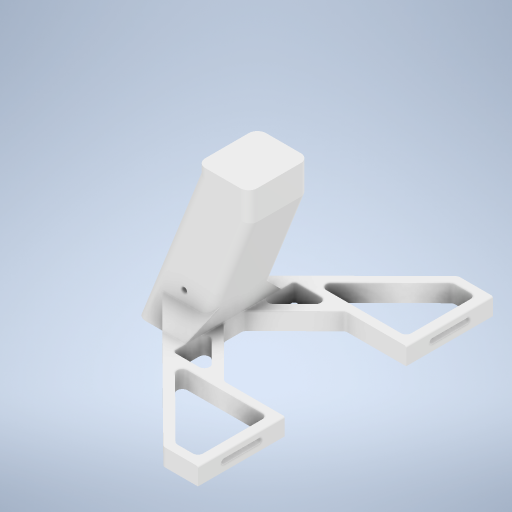
# Autodesk Inventor part: UpperLandingLegMount - BranchBrace+Shortened
Saved by Autodesk Inventor 2023 (Build 270158000, 158)
## iProperties
Created: 2023-01-11
Part Number: UpperLandingLegMount - BranchBrace+Shortened
Material: ABS Plastic
Document SubType Name: Modeling
Designer: chase
Density: 1.06 g/cm^3
Appearance: Smooth - White
Author: chase
Autodesk Inventor part; units mm, degrees
ref_plane "YZ Plane" through (0, 0, 0) normal (1, 0, 0) x (0, 1, 0)
ref_plane "XZ Plane" through (0, 0, 0) normal (0, 1, 0) x (-1, 0, 0)
ref_plane "XY Plane" through (0, 0, 0) normal (0, 0, 1) x (1, 0, 0)
sketch "Sketch1" plane through (0, 0, 0) normal (0, 0, 1) x (1, 0, 0)
  circle A0 centre (5.75, 0) radius 1.35 construction
  circle A1 centre (5.75, 0) radius 1.5
  circle A2 centre (24.25, 0) radius 1.55 construction
  circle A3 centre (24.25, 0) radius 1.5
  circle A4 centre (24.25, 22) radius 1.55 construction
  circle A5 centre (24.25, 22) radius 1.5
  circle A6 centre (5.75, 22) radius 1.35 construction
  circle A7 centre (5.75, 22) radius 1.5
  line L0 (5.75, 0) -> (0, 0) construction
  line L1 (0, 35.2322) -> (0, -14.7678) construction
  line L2 (5.75, 22) -> (24.25, 22) construction
  line L3 (24.25, 22) -> (24.25, 0) construction
  line L4 (24.25, 0) -> (5.75, 0) construction
  line L5 (5.75, 0) -> (5.75, 22) construction
  line L6 (0, -6.5) -> (30, -6.5)
  line L7 (30, -6.5) -> (30, 28.5)
  line L8 (30, 28.5) -> (0, 28.5)
  line L9 (0, 28.5) -> (0, -6.5)
  line L10 (30, 28.5) -> (30, 28.5)
  line L11 (30, 11) -> (0, 11) construction
  line L12 (0, 36) -> (5.124, 36)
  line L13 (0, -14) -> (5.124, -14)
  line L14 (0, 28.5) -> (0, 36)
  line L15 (5.124, 36) -> (23.4965, 67.8221)
  line L16 (5.124, -14) -> (23.4965, -45.8221)
  line L17 (16.6, 31.649) -> (16.6, 40.549)
  line L18 (16.6, 40.549) -> (18.8148, 40.549)
  line L19 (16.6, 31.649) -> (18.8148, 31.649)
  circle A8 centre (16.6, 40.549) radius 1.55
  circle A9 centre (16.6, 31.649) radius 1.55
  line L20 (16.6, -9.649) -> (16.6, -18.549)
  line L21 (16.6, -18.549) -> (18.8148, -18.549)
  line L22 (16.6, -9.649) -> (18.8148, -9.649)
  circle A10 centre (16.6, -18.549) radius 1.55
  circle A11 centre (16.6, -9.649) radius 1.55
  line L23 (23.4965, 67.8221) -> (28.6927, 64.8221)
  line L24 (16.6, 40.549) -> (16.6, 31.649) construction
  arc A12 (18.15, 40.549) -> (15.05, 40.549) centre (16.6, 40.549) ccw
  arc A13 (15.05, 31.649) -> (18.15, 31.649) centre (16.6, 31.649) ccw
  line L25 (28.6927, 64.8221) -> (23.9013, 28.5)
  line L26 (23.4965, -45.8221) -> (28.6927, -42.8221)
  line L27 (28.6927, -42.8221) -> (23.9013, -6.5)
  line L28 (0, -6.5) -> (0, -14)
  point P0 (0, 0)
  point P1 (0, 0)
  point P2 (16.6, -6.5)
  point P3 (16.6, -25.1317)
  point P4 (16.6, 36.099)
  dimension "d0" = 3
  dimension "d1" = 3
  dimension "d2" = 3
  dimension "d3" = 3
  dimension "d4" = 30
  dimension "d5" = 35
  dimension "d6" = 6.5
  dimension "d7" = 22
  dimension "d8" = 18.5
  dimension "d9" = 0
  dimension "d10" = 0
  dimension "d11" = 5.75
  dimension "d12" = 0
  dimension "d13" = 0
  dimension "d14" = 0
  dimension "d21" = 50
  dimension "d23" = 120
  dimension "d24" = 16.6
  dimension "d26" = 8.9
  dimension "d27" = 3.1
  dimension "d28" = 3.1
  dimension "d31" = 6
  constraints: 60 end point, 14 centre point, 9 symmetric about line, 7 coincident, 7 parallel, 5 point on line, 4 horizontal, 4 point on circle, 3 midpoint, 3 perpendicular, 2 collinear, 1 concentric, 1 vertical, 2 other
  measures "d0" diameter of A1
  measures "d1" diameter of A3
  measures "d2" diameter of A5
  measures "d3" diameter of A7
  measures "d4" distance of L9.end L7.start
  measures "d5" distance of L7.start L7.end
  measures "d6" distance from line of L6 A3.centre
  measures "d7" distance of L3.start L3.end
  measures "d8" distance of L3.end L5.start
  measures "d9" vertical distance of A3.centre A1.centre
  measures "d10" vertical distance of point (0, 0) A1.centre
  measures "d11" distance from line of L1 A1.centre
  measures "d12" horizontal distance of L5.end A1.centre
  measures "d13" distance from line of L1 point (0, 0)
  measures "d14" distance of L7.end L10.end
  measures "d21" distance between parallel lines of L12 L13
  measures "d23" angle of L12 L15
  measures "d24" distance between parallel lines of L14 L17
  measures "d26" distance between parallel lines of L18 L19
  measures "d27" diameter of A8
  measures "d28" diameter of A9
  measures "d31" distance of L15.end L23.end
extrude "Extrusion: MountFace" add sketch "Sketch1" against normal blind 5 contours A1 | A3 | A5 | A7 | L9 L8 L7 L6
draft "FaceDraft1" angle 21.5 pull direction (-1, 0, 0) fixed plane through (0, 16.8333, -1.6667) normal (-1, 0, 0) faces at (10, 16.8333, -5)
ref_plane "Work Plane: Vert" through (0, 11, 0) normal (0, 1, 0) x (1, 0, 0)
ref_plane "Work Plane: Brace" through (0, 0, -88.5) normal (0, 0, 1) x (1, 0, 0)
sketch "Sketch12" plane through (0, 0, -88.5) normal (0, 0, 1) x (1, 0, 0)
  line L0 (68.25, 96) -> (68.25, -74)
  ellipse E0 centre (-37.7144, 11) end of major axis (-37.7144, 22) minor radius 10.4013 (-30.7287, 2.8501) -> (-30.7287, 19.1499) ccw projected
  line L1 (68.25, 96) -> (48.25, 96)
  line L2 (48.25, 96) -> (48.25, -74)
  line L3 (48.25, -74) -> (68.25, -74)
  line L4 (68.25, -74) -> (68.25, 96)
  line L5 (-25.1358, -1.2423) -> (48.25, -74)
  line L6 (-25.1358, 23.2423) -> (48.25, 96)
  line L7 (53.25, -69) -> (63.25, -69)
  line L8 (63.25, -69) -> (63.25, 91)
  line L9 (63.25, 91) -> (53.25, 91)
  line L10 (53.25, 91) -> (53.25, -69)
  line L11 (-21.75, -4.5991) -> (-21.75, 26.5991)
  circle A0 centre (24.25, 22) radius 1.5 construction
  circle A1 centre (24.25, 22) radius 1.5 construction
  point P0 (0, 0)
  point P1 (-27.3131, 11)
  point P2 (63.25, 11)
  point P3 (68.25, 11)
  dimension "d91" = 170
  dimension "d92" = 85
  dimension "d95" = 20
  dimension "d106" = 0
  dimension "d111" = 10
  dimension "d112" = 160
  dimension "d115" = 70
  dimension "d117" = 0
  dimension "d161" = 44
  dimension "d162" = 5
  constraints: 24 end point, 4 parallel, 2 horizontal, 2 midpoint, 2 perpendicular, 2 point on line, 2 vertical, 2 vertical alignment, 1 centre point, 1 coincident, 4 other
  measures "d91" distance of L0.start L0.end
  measures "d92" vertical distance of point (-27.313, 11) L0.start
  measures "d95" distance of L3.end L2.end
  measures "d106" distance from line of L0.end L3
  measures "d111" distance of L9.end L8.end
  measures "d112" distance of L8.end L7.end
  measures "d115" distance between parallel lines of L2 L11
  measures "d117" vertical distance of point (68.25, 11) point (63.25, 11)
  measures "d161" distance from line of L4 A1.centre
  measures "d162" distance between parallel lines of L0 L8
extrude "Extrusion: Brace" add sketch "Sketch12" along normal mid plane 10 contours L0 L3 L2 L1 | L2 L5 L11 L6 | L10 L9 L8 L7
sketch "Sketch13" plane through (68.25, -74, -83.5) normal (1, 0, 0) x (0, 0, -1)
  line L0 (0, 0) -> (0, 170) construction
  line L1 (10, 100.5991) -> (10, 170) construction
  line L2 (0, 0) -> (10, 170) construction
  line L3 (5, 85) -> (5, 145)
  line L4 (5, 135) -> (5, 155) construction
  line L5 (6.55, 135) -> (6.55, 155)
  line L6 (3.45, 155) -> (3.45, 135)
  arc A0 (3.45, 135) -> (6.55, 135) centre (5, 135) ccw
  arc A1 (6.55, 155) -> (3.45, 155) centre (5, 155) ccw
  line L7 (5, 85) -> (5, 25)
  line L8 (5, 35) -> (5, 15) construction
  line L9 (3.45, 35) -> (3.45, 15)
  line L10 (6.55, 15) -> (6.55, 35)
  arc A2 (6.55, 35) -> (3.45, 35) centre (5, 35) ccw
  arc A3 (3.45, 15) -> (6.55, 15) centre (5, 15) ccw
  point P0 (-83.5, 74)
  point P1 (10, 97.4363)
  dimension "d98" = 60
  dimension "d99" = 10
  dimension "d100" = 3.1
  dimension "d101" = 60
  dimension "d102" = 10
  dimension "d103" = 3.1
  constraints: 22 end point, 8 point on circle, 8 tangent, 4 centre point, 4 vertical, 3 midpoint, 2 parallel
  measures "d98" distance of L3.start L3.end
  measures "d99" distance of L3.end L4.end
  measures "d100" diameter of A1
  measures "d101" distance of L3.start L7.end
  measures "d102" distance of L7.end L8.end
  measures "d103" diameter of A3
extrude "Extrusion: Slots" cut sketch "Sketch13" against normal blind 5
sketch "Sketch17" plane through (0, -6.5, -5) normal (-0.3665012, 0, -0.9304176) x (-0.9304176, 0, 0.3665012)
  line L0 (0, 0) -> (0, 35) projected
  line L1 (-32.2436, 0) -> (0, 0) projected
  line L2 (0, 35) -> (-32.2436, 35)
  line L3 (-32.2436, 35) -> (-32.2436, 0)
  line L4 (-32.2436, 0) -> (0, 0)
  line L5 (0, 0) -> (0, 35)
  point P0 (1.8325, 6.5)
  constraints: 8 end point, 2 parallel, 1 horizontal, 1 perpendicular
extrude "Extrusion: Pillar" add sketch "Sketch17" along normal blind 100
sketch "Sketch15" plane through (0, 0, -83.5) normal (0, 0, 1) x (1, 0, 0)
  line L0 (68.25, -74) -> (48.25, -74) projected
  line L1 (68.25, -74) -> (68.25, 96) projected
  line L2 (48.25, -74) -> (68.25, -74)
  line L3 (68.25, -74) -> (68.25, 96)
  line L4 (-21.75, -4.5991) -> (48.25, -74) projected
  line L5 (48.25, -74) -> (-21.75, -4.5991)
  line L6 (-30.3821, 11) -> (50.3085, -69)
  line L7 (50.3085, -69) -> (63.25, -69)
  line L8 (63.25, -69) -> (63.25, 101)
  line L9 (-30.3821, 11) -> (50.3085, 91)
  line L10 (48.25, 96) -> (-21.75, 26.5991) projected
  line L11 (50.3085, 91) -> (63.25, 91)
  line L12 (68.25, 96) -> (48.25, 96) projected
  line L13 (63.25, -69) -> (58.25, -69)
  line L14 (58.25, -69) -> (58.25, -29)
  line L15 (58.25, -29) -> (63.25, -29)
  line L16 (63.25, -29) -> (63.25, -69)
  line L17 (63.25, 91) -> (58.25, 91)
  line L18 (58.25, 91) -> (58.25, 51)
  line L19 (58.25, 51) -> (63.25, 51)
  line L20 (63.25, 51) -> (63.25, 91)
  line L21 (58.25, -29) -> (9.9632, -29)
  line L22 (4.92, -24) -> (63.25, -24)
  line L23 (4.92, 46) -> (63.25, 46)
  line L24 (9.9632, 51) -> (58.25, 51)
  line L25 (-19.8327, 28.5) -> (48.25, 96) projected
  line L26 (48.25, 96) -> (68.25, 96) projected
  line L27 (68.25, 96) -> (68.25, -74) projected
  line L28 (68.25, -74) -> (48.25, -74) projected
  line L29 (48.25, -74) -> (-19.8327, -6.5) projected
  line L30 (3.733, -6.5) -> (-19.8327, -6.5) projected
  line L31 (3.733, 28.5) -> (3.733, -6.5) projected
  line L32 (-19.8327, 28.5) -> (3.733, 28.5) projected
  line L33 (-30.922, 28.5) -> (-19.8327, 28.5) projected
  line L34 (-30.922, -6.5) -> (-30.922, 28.5) projected
  line L35 (-19.8327, -6.5) -> (-30.922, -6.5) projected
  line L36 (-19.8327, 28.5) -> (3.733, 28.5) projected
  line L37 (63.25, -24) -> (68.25, -24)
  line L38 (63.25, 46) -> (68.25, 46)
  line L39 (3.733, 28.5) -> (3.733, -6.5) projected
  line L40 (-0.2061, -6.5) -> (-0.2061, 28.5) projected
  line L41 (26.225, -24) -> (2.9389, -0.9132)
  line L42 (3.733, 23.7005) -> (26.225, 46)
  line L43 (33.3266, -24) -> (3.733, 5.3404)
  line L44 (3.733, 16.6596) -> (33.3266, 46)
  line L45 (3.733, -6.5) -> (3.733, 28.5)
  line L46 (3.733, -6.5) -> (-19.8327, -6.5) projected
  line L47 (3.733, -6.5) -> (3.733, -22.8231)
  line L48 (3.733, 28.5) -> (3.733, 44.8231)
  line L49 (3.733, -22.8231) -> (3.733, 44.8231)
  point P0 (0, 0)
  point P1 (34.1066, 51)
  point P2 (63.25, 51)
  point P3 (63.25, -29)
  point P4 (3.733, 16.8663)
  point P5 (68.25, 46)
  point P6 (68.25, -24)
  point P7 (14.582, -12.4566)
  point P8 (14.979, 34.8503)
  point P9 (3.733, -1.7005)
  point P10 (4.2872, 4.7909)
  point P11 (-12.731, -6.5)
  point P12 (3.733, 23.7005)
  point P13 (3.733, -6.5)
  dimension "d119" = 5
  dimension "d120" = 5
  dimension "d121" = 5
  dimension "d122" = 5
  dimension "d123" = 5
  dimension "d124" = 5
  dimension "d125" = 40
  dimension "d126" = 40
  dimension "d127" = 5
  dimension "d128" = 5
  dimension "d157" = 15
  dimension "d158" = 15
  dimension "d159" = 5
  dimension "d160" = 5
  constraints: 60 end point, 18 point on line, 12 parallel, 8 horizontal, 5 midpoint, 4 perpendicular, 4 vertical, 2 coincident, 2 collinear, 2 other
  measures "d119" distance between parallel lines of L4 L6
  measures "d120" distance between parallel lines of L2 L7
  measures "d121" distance between parallel lines of L1 L8
  measures "d122" distance between parallel lines of L10 L9
  measures "d124" distance of L14.end L15.end
  measures "d125" distance of L13.end L14.end
  measures "d126" distance of L18.end L17.end
  measures "d127" distance between parallel lines of L22 L21
  measures "d128" distance from line of point (34.107, 51) L23
  measures "d157" distance from line of point (14.582, -12.457) L6
  measures "d158" distance from line of L9 point (14.979, 34.85)
  measures "d159" distance between parallel lines of L41 L43
  measures "d160" distance between parallel lines of L42 L44
extrude "Extrusion: Lightening" cut sketch "Sketch15" against normal up to surface (10 mm away) contours L37 L8 L38 L1 | L22 L43 L31 L44 L23 L8 | L8 L7 L14 L15 | L47 L31 L41 L22 L6 | L19 L18 L11 L8 | L14 L7 L6 L21 | L24 L9 L11 L18 | L42 L31 L48 L9 L23
sketch "Sketch16" plane through (0, 0, -93.5) normal (0, 0, -1) x (-1, 0, 0)
  line L0 (65.3576, 48.2147) -> (-32.3626, 48.2147)
  line L1 (-32.3626, 48.2147) -> (-32.3626, -28.742)
  line L2 (-32.3626, -28.742) -> (65.3576, -28.742)
  line L3 (65.3576, -28.742) -> (65.3576, 48.2147)
  point P0 (0, 0)
  constraints: 8 end point, 2 parallel, 1 horizontal, 1 perpendicular
extrude "Extrusion: RemoveBot" cut sketch "Sketch16" along normal through all
sketch "Sketch19" plane through (0, -6.5, 0) normal (0, -1, 0) x (1, 0, 0)
  line L0 (0, -5) -> (-34.8611, -93.5) construction
  line L1 (-22.0783, -61.0491) -> (7.9217, -72.8664) construction
  line L2 (30, -16.8173) -> (3.733, -83.5) construction
  circle A0 centre (-7.0783, -66.9578) radius 1.5
  point P0 (0, 0)
  point P1 (3.733, -83.5)
  point P2 (2.9389, -83.5)
  point P3 (3.733, -83.5)
  dimension "d140" = 3
  constraints: 2 end point, 1 centre point, 1 midpoint, 1 point on line, 2 other
  measures "d140" diameter of A0
extrude "Extrusion: Pin" cut sketch "Sketch19" against normal up to surface (35 mm away)
chamfer "Chamfer: PillarSupport" distance 10 angle 45 2 edges at (-8.0499, -6.5, -83.5) (-8.0499, 28.5, -83.5)
fillet "Fillet: Pillar" radius 5 8 edges at (-17.4305, 28.5, -49.25) (-17.4305, -6.5, -49.25) (0, 28.5, -2.5) (0, -6.5, -2.5) (18.836, 28.5, -45.1587) (18.836, -6.5, -45.1587) (30, -6.5, -8.4087) (30, 28.5, -8.4087)
fillet "Fillet: SlotLip" radius 1 2 edges at (68.25, 71, -83.5) (68.25, -49, -83.5)
fillet "Fillet: 3mmCorners" radius 3 18 edges at (9.9632, -29, -88.5) (9.9632, 51, -88.5) (50.3085, -69, -88.5) (50.3085, 91, -88.5) (48.25, 96, -88.5) (48.25, -74, -88.5) (26.225, -24, -88.5) (3.733, -1.7005, -88.5) (3.733, 23.7005, -88.5) (26.225, 46, -88.5) (63.25, -29, -88.5) (63.25, -69, -88.5) (63.25, 51, -88.5) (63.25, 91, -88.5) (3.733, 5.3404, -88.5) (3.733, 16.6596, -88.5) (33.3266, 46, -88.5) (33.3266, -24, -88.5)
ref_plane "Work Plane: OffsetFromFaceDraft" through (11.6749, -6.5, -63.3382) normal (-0.3665012, 0, -0.9304176) x (-0.9304176, 0, 0.3665012)
ref_plane "Work Plane: FaceDraft" through (30, -6.5, -16.8173) normal (-0.3665012, 0, -0.9304176) x (-0.9304176, 0, 0.3665012)
sketch "Sketch21" plane through (11.6749, -6.5, -63.3382) normal (-0.3665012, 0, -0.9304176) x (-0.9304176, 0, 0.3665012)
  arc A0 (27.2436, 0) -> (32.2436, 5) centre (27.2436, 5) ccw construction
  arc A1 (5, 35) -> (0, 30) centre (5, 30) ccw construction
  line L0 (27.2436, 0) -> (5, 35) construction
  circle A2 centre (16.1218, 17.5) radius 8.125
  point P0 (34.0761, 6.5)
  dimension "d169" = 16.25
  constraints: 2 end point, 1 centre point, 1 midpoint
  measures "d169" diameter of A2
extrude "Extrusion18" cut sketch "Sketch21" along normal through all
ref_plane "Work Plane: Mid" through (-19.8327, 11, -93.5) normal (0, -1, 0) x (1, 0, 0)
ref_plane "Work Plane13" through (5.75, -1.5, 0) normal (-1, 0, 0) x (0, 0, 1)
sketch "Sketch: LegOverallGeometry" plane through (-19.8327, 11, -93.5) normal (0, -1, 0) x (1, 0, 0)
  line L0 (24.8327, 87.5507) -> (19.8327, 88.5) construction
  line L1 (19.8327, 88.5) -> (49.8327, 88.5) construction
  line L2 (49.8327, 93.5) -> (49.8327, 76.6827) construction
  line L3 (24.0827, 93.5) -> (27.0827, 93.5) construction
  line L4 (25.5827, 93.5) -> (25.5827, 88.5) construction
  line L5 (19.8327, 88.5) -> (19.8327, -287.5) construction
  line L6 (19.8327, -287.5) -> (38.3327, -287.5) construction
  line L7 (38.3327, -287.5) -> (186.3327, -287.5) construction
  line L8 (112.3327, -287.5) -> (-116.2673, -287.5) construction
  line L9 (112.3327, -287.5) -> (340.9327, -287.5) construction
  line L10 (112.3327, -287.5) -> (112.3327, 93.5) construction
  line L11 (112.3327, 93.5) -> (312.3327, 93.5) construction
  line L12 (112.3327, 93.5) -> (-87.6673, 93.5) construction
  line L13 (-116.2673, -287.5) -> (39.3327, 93.5) construction
  line L14 (340.9327, -287.5) -> (185.3327, 93.5) construction
  line L15 (39.3327, 93.5) -> (39.3327, -19.4487) construction
  line L16 (49.8327, 76.6827) -> (44.8327, 77.632) construction
  line L17 (19.8327, 88.5) -> (49.8327, 76.6827) construction
  point P0 (19.8327, 93.5)
  dimension "d175" = 18.5
  dimension "d176" = 148
  dimension "d177" = 228.6
  dimension "d179" = 381
  dimension "d180" = 228.6
  dimension "d182" = 200
  dimension "d183" = 200
  dimension "d184" = 381
  dimension "d185" = 73
  dimension "d186" = 73
  dimension "d189" = 22.215
  constraints: 28 end point, 6 horizontal, 5 point on line, 3 vertical, 2 midpoint, 1 coincident, 1 perpendicular
  measures "d175" distance of L5.end L6.end
  measures "d176" distance of L6.end L7.end
  measures "d177" distance of L8.start L8.end
  measures "d179" distance of point (19.833, 93.5) L5.end
  measures "d180" distance of L8.start L9.end
  measures "d182" distance of L10.end L11.end
  measures "d183" distance of L10.end L12.end
  measures "d184" distance of L8.start L10.end
  measures "d185" distance of L14.end L10.end
  measures "d186" distance of L10.end L13.end
  measures "d189" angle of L15 L13
equation "\"d6\" = -0.5 * d7 + 0.5 * d5"
equation "\"d11\" = -0.5 * d8 + 0.5 * d4"
equation "\"d92\" = 0.5 * d91"
body "Solid1"
